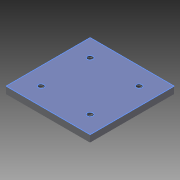
# Autodesk Inventor part: Base Plate
Saved by Autodesk Inventor 2016 (Build 200138000, 138)
## iProperties
Created: 2014-03-06
Part Number: Base Plate
Material: Aluminum 6061
Document SubType Name: Modeling
Designer: John
Density: 1 g/cm^3
Appearance: Aluminum - Flat
Author: John
Autodesk Inventor part; units mm, degrees
ref_plane "YZ Plane" through (0, 0, 0) normal (1, 0, 0) x (0, 1, 0)
ref_plane "XZ Plane" through (0, 0, 0) normal (0, 1, 0) x (-1, 0, 0)
ref_plane "XY Plane" through (0, 0, 0) normal (0, 0, 1) x (1, 0, 0)
sketch "Sketch1" plane through (0, 0, 0) normal (0, 1, 0) x (-1, 0, 0)
  line L0 (38.1, -38.1) -> (-38.1, -38.1)
  line L1 (-38.1, -38.1) -> (-38.1, 38.1)
  line L2 (-38.1, 38.1) -> (38.1, 38.1)
  line L3 (38.1, 38.1) -> (38.1, -38.1)
  line L4 (38.1, -38.1) -> (-38.1, 38.1) construction
  line L5 (-38.1, -38.1) -> (38.1, 38.1) construction
  point P0 (0, 0)
  dimension "d0" = 76.2
  dimension "d1" = 76.2
  constraints: 12 end point, 2 midpoint, 2 parallel, 1 horizontal, 1 perpendicular
  measures "d0" distance of L1.end L2.end
  measures "d1" distance of L0.end L1.end
extrude "Extrusion1" add sketch "Sketch1" along normal blind 6.35
sketch "Sketch2" plane through (0, 6.35, 0) normal (0, 1, 0) x (1, 0, 0)
  line L0 (38.1, 38.1) -> (-38.1, 38.1) projected
  line L1 (-38.1, 38.1) -> (-38.1, -38.1) projected
  line L2 (-38.1, -38.1) -> (38.1, -38.1) projected
  line L3 (38.1, -38.1) -> (38.1, 38.1) projected
  line L4 (-22.225, 22.225) -> (22.225, 22.225)
  line L5 (22.225, 22.225) -> (22.225, -22.225)
  line L6 (22.225, -22.225) -> (-22.225, -22.225)
  line L7 (-22.225, -22.225) -> (-22.225, 22.225)
  point P0 (0, 0)
  dimension "d4" = 15.875
  constraints: 8 end point, 3 other
  measures "d4" distance between parallel lines of L0 L4
hole "Hole1" at (-22.225, 6.35, -22.225) at (22.225, 6.35, 22.225) at (22.225, 6.35, -22.225) at (-22.225, 6.35, 22.225) direction (0, -1, 0) diameter 4.9784 end through all thread size "1/4-20 UNC" class "2B" standard "ANSI Unified Screw Threads"
body "Solid1"
